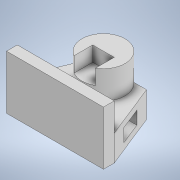
# Autodesk Inventor part: Część3
Saved by Autodesk Inventor 2021 (Build 250183000, 183)
## iProperties
Created: 2024-05-10
Part Number: Część3
Material: Ogólny
Document SubType Name: Modeling
Designer: Dawidek
Density: 1 g/cm^3
Appearance: Domyślna
Author: Dawidek
Autodesk Inventor part; units mm, degrees
ref_plane "YZ Plane" through (0, 0, 0) normal (1, 0, 0) x (0, 1, 0)
ref_plane "XZ Plane" through (0, 0, 0) normal (0, 1, 0) x (-1, 0, 0)
ref_plane "XY Plane" through (0, 0, 0) normal (0, 0, 1) x (1, 0, 0)
sketch "Szkic1" plane through (0, 0, 0) normal (0, 0, 1) x (1, 0, 0)
  line L0 (0, 0) -> (90, 0)
  line L1 (90, 0) -> (90, 50)
  line L2 (90, 50) -> (0, 50)
  line L3 (0, 50) -> (0, 0)
  dimension "d0" = 90
  dimension "d1" = 50
  constraints: 8 end point, 3 perpendicular, 1 horizontal
  measures "d0" distance of L0.start L0.end
  measures "d1" distance of L0.end L1.end
extrude "Wyciągnięcie proste1" add sketch "Szkic1" along normal blind 10
sketch "Szkic2" plane through (0, 0, 0) normal (0, -1, 0) x (1, 0, 0)
  line L0 (90, 0) -> (0, 0) projected
  line L1 (20, -50) -> (70, -50)
  line L2 (70, -50) -> (90, 0)
  line L3 (90, 0) -> (0, 0)
  line L4 (0, 0) -> (0, 10) projected
  line L5 (20, -50) -> (0, 0)
  line L6 (0, 0) -> (90, 0)
  dimension "d6" = 50
  constraints: 10 end point, 1 collinear, 1 horizontal
  measures "d6" distance of L1.start L1.end
extrude "Wyciągnięcie proste2" add sketch "Szkic2" against normal blind 24
sketch "Szkic3" plane through (0, 24, 0) normal (0, 1, 0) x (1, 0, 0)
  line L0 (0, 0) -> (0, -10) projected
  line L1 (90, 0) -> (0, 0) projected
  circle A0 centre (45, 35) radius 20
  dimension "d11" = 40
  constraints: 1 centre point
  measures "d11" diameter of A0
extrude "Wyciągnięcie proste3" add sketch "Szkic3" along normal blind 26
sketch "Szkic4" plane through (0, 0, 10) normal (0, -1, 0) x (1, 0, 0)
  line L0 (70, -60) -> (58.2288, -60) projected
  line L1 (70, -60) -> (70, -66.9782)
  line L2 (70, -66.9782) -> (20, -66.9782)
  line L3 (31.7712, -60) -> (20, -60) projected
  line L4 (20, -66.9782) -> (20, -60)
  line L5 (20, -60) -> (70, -60)
  point P0 (0, -10)
  constraints: 8 end point, 3 perpendicular, 1 vertical
extrude "Wyciągnięcie proste4" cut sketch "Szkic4" against normal blind 35
sketch "Szkic5" plane through (0, 0, 10) normal (-1, 0, 0) x (0, 0, 1)
  line L0 (-25, 6) -> (-25, 18)
  line L1 (-25, 18) -> (-45, 18)
  line L2 (-45, 18) -> (-45, 6)
  line L3 (-45, 6) -> (-25, 6)
  point P0 (-10, 0)
  dimension "d18" = 12
  dimension "d19" = 20
  constraints: 8 end point, 3 perpendicular
  measures "d18" distance of L0.start L0.end
  measures "d19" distance of L0.end L1.end
extrude "Wyciągnięcie proste5" cut sketch "Szkic5" against normal blind 95
sketch "Szkic6" plane through (45, 50, -35) normal (0, 1, 0) x (1, 0, 0)
  line L0 (-31, 0) -> (31, 0) projected
  line L1 (0, 0) -> (10, 0)
  line L2 (10, 0) -> (10, -28.0711)
  line L3 (10, -28.0711) -> (-10, -28.0711)
  line L4 (-10, -28.0711) -> (-10, 0)
  line L5 (-10, 0) -> (0, 0)
  point P0 (-45, -35)
  dimension "d22" = 10
  dimension "d23" = 20
  constraints: 10 end point, 3 perpendicular, 2 point on line, 1 collinear, 1 midpoint
  measures "d22" distance of L1.start L1.end
  measures "d23" distance of L2.end L3.end
extrude "Wyciągnięcie proste6" cut sketch "Szkic6" against normal blind 14
